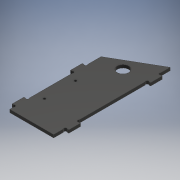
# Autodesk Inventor part: BA23
Saved by Autodesk Inventor 2017 (Build 210142000, 142)
## iProperties
Created: 2019-06-06
Part Number: BA23
Material: Polyethylene, High Density
Document SubType Name: Modeling
Designer: Dell
Density: 0.952 g/cm^3
Appearance: Smooth - Black
Author: Dell
Autodesk Inventor part; units mm, degrees
ref_plane "YZ Plane" through (0, 0, 0) normal (1, 0, 0) x (0, 1, 0)
ref_plane "XZ Plane" through (0, 0, 0) normal (0, 1, 0) x (-1, 0, 0)
ref_plane "XY Plane" through (0, 0, 0) normal (0, 0, 1) x (1, 0, 0)
sketch "Sketch1" plane through (0, 0, 0) normal (0, 0, 1) x (1, 0, 0)
  line L0 (0, 0) -> (95.25, 0)
  line L1 (95.25, 0) -> (95.25, 198.2931)
  line L2 (95.25, 198.2931) -> (0, 198.2931)
  line L3 (0, 198.2931) -> (0, 0)
  line L4 (0, 198.2931) -> (95.25, 253.2857)
  line L5 (95.25, 253.2857) -> (95.25, 198.2646)
  dimension "d0" = 95.25
  dimension "d1" = 198.293
  dimension "d2" = 60
  constraints: 12 end point, 2 parallel, 1 horizontal, 1 perpendicular, 1 point on line, 1 vertical
  measures "d0" distance of L2.end L1.end
  measures "d1" distance of L0.end L1.end
  measures "d2" angle of L5 L4
extrude "Extrusion1" add sketch "Sketch1" along normal blind 6.35
sketch "Sketch2" plane through (0, 0, 6.35) normal (0, 0, 1) x (1, 0, 0)
  line L0 (0, 198.2931) -> (0, 0) projected
  line L1 (0, 38.1146) -> (-7.62, 38.1146)
  line L2 (-7.62, 38.1146) -> (-7.62, 12.7146)
  line L3 (-7.62, 12.7146) -> (0, 12.7146)
  line L4 (0, 12.7146) -> (0, 38.1146)
  line L5 (0, 165.1146) -> (-7.62, 165.1146)
  line L6 (-7.62, 165.1146) -> (-7.62, 139.7146)
  line L7 (-7.62, 139.7146) -> (0, 139.7146)
  line L8 (0, 139.7146) -> (0, 165.1146)
  line L9 (0, 0) -> (95.25, 0) projected
  dimension "d5" = 7.62
  dimension "d6" = 25.4
  dimension "d7" = 25.4
  dimension "d8" = 101.6
  dimension "d9" = 12.7146
  constraints: 16 end point, 4 parallel, 2 horizontal, 2 perpendicular, 2 point on line, 1 vertical alignment
  measures "d5" distance of L3.end L2.end
  measures "d6" distance of L2.end L1.end
  measures "d7" distance of L5.end L6.end
  measures "d8" distance between parallel lines of L1 L7
  measures "d9" distance between parallel lines of L9 L3
extrude "Extrusion2" add sketch "Sketch2" against normal blind 6.35
sketch "Sketch3" plane through (0, 0, 6.35) normal (0, 0, 1) x (1, 0, 0)
  line L0 (95.25, 0) -> (95.25, 253.2857) projected
  line L1 (95.25, 228.6) -> (102.87, 228.6)
  line L2 (102.87, 228.6) -> (102.87, 203.2)
  line L3 (102.87, 203.2) -> (95.25, 203.2)
  line L4 (95.25, 203.2) -> (95.25, 228.6)
  line L5 (95.25, 50.8) -> (102.87, 50.8)
  line L6 (102.87, 50.8) -> (102.87, 25.4)
  line L7 (102.87, 25.4) -> (95.25, 25.4)
  line L8 (95.25, 25.4) -> (95.25, 50.8)
  line L9 (102.87, 215.9) -> (102.87, 38.1) construction
  line L10 (0, 0) -> (95.25, 0) projected
  point P0 (102.87, 127)
  point P1 (95.25, 126.6428)
  dimension "d13" = 25.4
  dimension "d14" = 7.62
  dimension "d15" = 25.4
  dimension "d16" = 177.8
  dimension "d19" = 25.4
  constraints: 18 end point, 4 midpoint, 4 parallel, 2 horizontal, 2 perpendicular, 2 point on line, 1 vertical
  measures "d13" distance of L1.end L2.end
  measures "d14" distance of L6.end L7.end
  measures "d15" distance of L5.end L6.end
  measures "d16" distance of L9.start L9.end
  measures "d19" distance between parallel lines of L10 L7
extrude "Extrusion3" add sketch "Sketch3" against normal blind 6.35
sketch "Sketch4" plane through (0, 0, 6.35) normal (0, 0, 1) x (1, 0, 0)
  circle A0 centre (17.7, 124.9622) radius 2.5
  circle A1 centre (17.7, 57.4622) radius 2.5
  line L0 (0, 139.7146) -> (0, 38.1146) projected
  line L1 (0, 0) -> (95.25, 0) projected
  dimension "d20" = 5
  dimension "d21" = 5
  dimension "d22" = 17.7
  dimension "d23" = 67.5
  dimension "d24" = 57.4622
  constraints: 2 centre point, 1 vertical alignment
  measures "d20" diameter of A0
  measures "d21" diameter of A1
  measures "d22" distance from line of L0 A0.centre
  measures "d23" distance of A1.centre A0.centre
  measures "d24" distance from line of L1 A1.centre
extrude "Extrusion4" cut sketch "Sketch4" against normal through all
sketch "Sketch5" plane through (0, 0, 6.35) normal (0, 0, 1) x (1, 0, 0)
  circle A0 centre (47.625, 198.2931) radius 12.5
  line L0 (0, 0) -> (95.25, 0) projected
  point P0 (0, 198.2931)
  point P1 (47.625, 0)
  dimension "d27" = 25
  constraints: 1 centre point, 1 horizontal alignment, 1 midpoint, 1 vertical alignment
  measures "d27" diameter of A0
extrude "Extrusion5" cut sketch "Sketch5" against normal through all
sketch "Sketch6" plane through (0, 0, 6.35) normal (0, 0, 1) x (1, 0, 0)
  circle A0 centre (47.625, 198.2931) radius 12.5 construction
  circle A1 centre (17.7, 124.9622) radius 2.5 construction
  circle A2 centre (17.7, 57.4622) radius 2.5 construction
  line L0 (95.25, 0) -> (95.25, 25.4) construction
  line L1 (95.25, 25.4) -> (102.87, 25.4) construction
  line L2 (102.87, 25.4) -> (102.87, 50.8) construction
  line L3 (102.87, 50.8) -> (95.25, 50.8) construction
  line L4 (95.25, 50.8) -> (95.25, 203.2) construction
  line L5 (95.25, 203.2) -> (102.87, 203.2) construction
  line L6 (102.87, 203.2) -> (102.87, 228.6) construction
  line L7 (102.87, 228.6) -> (95.25, 228.6) construction
  line L8 (95.25, 228.6) -> (95.25, 253.2857) construction
  line L9 (95.25, 253.2857) -> (0, 198.2931) construction
  line L10 (0, 198.2931) -> (0, 165.1146) construction
  line L11 (0, 165.1146) -> (-7.62, 165.1146) construction
  line L12 (-7.62, 165.1146) -> (-7.62, 139.7146) construction
  line L13 (-7.62, 139.7146) -> (0, 139.7146) construction
  line L14 (0, 139.7146) -> (0, 38.1146) construction
  line L15 (0, 38.1146) -> (-7.62, 38.1146) construction
  line L16 (-7.62, 38.1146) -> (-7.62, 12.7146) construction
  line L17 (-7.62, 12.7146) -> (0, 12.7146) construction
  line L18 (0, 12.7146) -> (0, 0) construction
  line L19 (0, 0) -> (95.25, 0) construction
  line L20 (-2.2451, 167.3597) -> (-2.2451, 199.5892) construction
  line L21 (-2.2451, 199.5892) -> (97.4951, 257.1742) construction
  line L22 (97.4951, 257.1742) -> (97.4951, 230.8451) construction
  line L23 (97.4951, 230.8451) -> (105.1151, 230.8451) construction
  line L24 (105.1151, 230.8451) -> (105.1151, 200.9549) construction
  line L25 (105.1151, 200.9549) -> (97.4951, 200.9549) construction
  line L26 (97.4951, 200.9549) -> (97.4951, 53.0451) construction
  line L27 (97.4951, 53.0451) -> (105.1151, 53.0451) construction
  line L28 (105.1151, 53.0451) -> (105.1151, 23.1549) construction
  line L29 (105.1151, 23.1549) -> (97.4951, 23.1549) construction
  line L30 (97.4951, 23.1549) -> (97.4951, -2.2451) construction
  line L31 (97.4951, -2.2451) -> (-2.2451, -2.2451) construction
  line L32 (-2.2451, -2.2451) -> (-2.2451, 10.4695) construction
  line L33 (-2.2451, 10.4695) -> (-9.8651, 10.4695) construction
  line L34 (-9.8651, 10.4695) -> (-9.8651, 40.3597) construction
  line L35 (-9.8651, 40.3597) -> (-2.2451, 40.3597) construction
  line L36 (-2.2451, 40.3597) -> (-2.2451, 137.4695) construction
  line L37 (-2.2451, 137.4695) -> (-9.8651, 137.4695) construction
  line L38 (-9.8651, 137.4695) -> (-9.8651, 167.3597) construction
  line L39 (-9.8651, 167.3597) -> (-2.2451, 167.3597) construction
  circle A3 centre (97.4951, 230.8451) radius 3.175
  line L40 (95.25, 50.8) -> (95.25, 203.2) projected
  circle A4 centre (97.4951, 200.9549) radius 3.175
  circle A5 centre (97.4951, 53.0451) radius 3.175
  circle A6 centre (97.4951, 23.1549) radius 3.175
  line L41 (0, 12.7146) -> (0, 0) projected
  circle A7 centre (-2.2451, 10.4695) radius 3.175
  line L42 (0, 139.7146) -> (0, 38.1146) projected
  circle A8 centre (-2.2451, 40.3597) radius 3.175
  circle A9 centre (-2.2451, 137.4695) radius 3.175
  line L43 (0, 198.2931) -> (0, 165.1146) projected
  circle A10 centre (-2.2451, 167.3597) radius 3.175
  dimension "d30" = 6.35
  constraints: 40 end point, 8 coincident, 43 other
extrude "Extrusion6" cut sketch "Sketch6" against normal through all
equation "\"d3\" = Panel_Thickness"
equation "\"d5\" = Panel_Thickness + Fit_Tolerance"
equation "\"d10\" = Panel_Thickness"
equation "\"d14\" = Panel_Thickness + Fit_Tolerance"
equation "\"d17\" = Panel_Thickness"
equation "\"d25\" = Panel_Thickness"
equation "\"d28\" = Panel_Thickness"
equation "\"d30\" = Tool_Dia"
equation "\"d31\" = Panel_Thickness"
equation "\"Panel_Thickness\" = 6.35"
equation "\"Fit_Tolerance\" = 1.27"
equation "\"Tool_Dia\" = 6.35"
body "Solid1"
